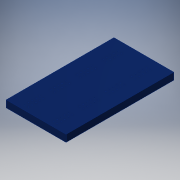
# Autodesk Inventor part: Assembly Plate
Saved by Autodesk Inventor 2019.4 (Build 234330000, 330)
## iProperties
Created: 2021-01-11
Part Number: Assembly Plate
Material: Aluminum, Anodized Blue
Document SubType Name: Modeling
Designer: caleb
Density: 2.7 g/cm^3
Appearance: Anodized - Blue
Author: caleb
Autodesk Inventor part; units mm, degrees
ref_plane "YZ Plane" through (0, 0, 0) normal (1, 0, 0) x (0, 1, 0)
ref_plane "XZ Plane" through (0, 0, 0) normal (0, 1, 0) x (-1, 0, 0)
ref_plane "XY Plane" through (0, 0, 0) normal (0, 0, 1) x (1, 0, 0)
sketch "Sketch1" plane through (0, 0, 0) normal (0, 1, 0) x (-1, 0, 0)
  line L0 (-60, 108) -> (60, 108)
  line L1 (60, 108) -> (60, -108)
  line L2 (60, -108) -> (-60, -108)
  line L3 (-60, -108) -> (-60, 108)
  line L4 (-60, 108) -> (60, -108) construction
  line L5 (60, 108) -> (-60, -108) construction
  point P0 (0, 0)
  dimension "d0" = 120
  dimension "d1" = 216
  constraints: 12 end point, 2 midpoint, 2 parallel, 1 horizontal, 1 perpendicular
  measures "d0" distance of L1.end L2.end
  measures "d1" distance of L0.end L1.end
extrude "Extrusion1" add sketch "Sketch1" along normal blind 14
sketch "Sketch4" plane through (0, 14, 0) normal (0, 1, 0) x (1, 0, 0)
  circle A0 centre (-32.57, -98.05) radius 0.75
  line L0 (-60, 108) -> (-60, -108) projected
  line L1 (-60, -108) -> (60, -108) projected
  circle A1 centre (-32.57, -90.62) radius 0.75
  circle A2 centre (-32.57, -83.19) radius 0.75
  circle A3 centre (-32.57, -75.76) radius 0.75
  circle A4 centre (-32.57, -68.33) radius 0.75
  circle A5 centre (-25.14, -98.05) radius 0.75
  circle A6 centre (-25.14, -90.62) radius 0.75
  circle A7 centre (-25.14, -83.19) radius 0.75
  circle A8 centre (-25.14, -75.76) radius 0.75
  circle A9 centre (-25.14, -68.33) radius 0.75
  circle A10 centre (-32.57, -45.85) radius 0.75
  circle A11 centre (-32.57, -38.42) radius 0.75
  circle A12 centre (-32.57, -30.99) radius 0.75
  circle A13 centre (-32.57, -23.56) radius 0.75
  circle A14 centre (-32.57, -16.13) radius 0.75
  circle A15 centre (-25.14, -45.85) radius 0.75
  circle A16 centre (-25.14, -38.42) radius 0.75
  circle A17 centre (-25.14, -30.99) radius 0.75
  circle A18 centre (-25.14, -23.56) radius 0.75
  circle A19 centre (-25.14, -16.13) radius 0.75
  circle A20 centre (-32.57, 6.35) radius 0.75
  circle A21 centre (-32.57, 13.78) radius 0.75
  circle A22 centre (-32.57, 21.21) radius 0.75
  circle A23 centre (-32.57, 28.64) radius 0.75
  circle A24 centre (-32.57, 36.07) radius 0.75
  circle A25 centre (-25.14, 6.35) radius 0.75
  circle A26 centre (-25.14, 13.78) radius 0.75
  circle A27 centre (-25.14, 21.21) radius 0.75
  circle A28 centre (-25.14, 28.64) radius 0.75
  circle A29 centre (-25.14, 36.07) radius 0.75
  circle A30 centre (-32.57, 58.55) radius 0.75
  circle A31 centre (-32.57, 65.98) radius 0.75
  circle A32 centre (-32.57, 73.41) radius 0.75
  circle A33 centre (-32.57, 80.84) radius 0.75
  circle A34 centre (-32.57, 88.27) radius 0.75
  circle A35 centre (-25.14, 58.55) radius 0.75
  circle A36 centre (-25.14, 65.98) radius 0.75
  circle A37 centre (-25.14, 73.41) radius 0.75
  circle A38 centre (-25.14, 80.84) radius 0.75
  circle A39 centre (-25.14, 88.27) radius 0.75
  circle A40 centre (25.14, -98.05) radius 0.75
  circle A41 centre (25.14, -90.62) radius 0.75
  circle A42 centre (25.14, -83.19) radius 0.75
  circle A43 centre (25.14, -75.76) radius 0.75
  circle A44 centre (25.14, -68.33) radius 0.75
  circle A45 centre (32.57, -98.05) radius 0.75
  circle A46 centre (32.57, -90.62) radius 0.75
  circle A47 centre (32.57, -83.19) radius 0.75
  circle A48 centre (32.57, -75.76) radius 0.75
  circle A49 centre (32.57, -68.33) radius 0.75
  circle A50 centre (25.14, -45.85) radius 0.75
  circle A51 centre (25.14, -38.42) radius 0.75
  circle A52 centre (25.14, -30.99) radius 0.75
  circle A53 centre (25.14, -23.56) radius 0.75
  circle A54 centre (25.14, -16.13) radius 0.75
  circle A55 centre (32.57, -45.85) radius 0.75
  circle A56 centre (32.57, -38.42) radius 0.75
  circle A57 centre (32.57, -30.99) radius 0.75
  circle A58 centre (32.57, -23.56) radius 0.75
  circle A59 centre (32.57, -16.13) radius 0.75
  circle A60 centre (25.14, 6.35) radius 0.75
  circle A61 centre (25.14, 13.78) radius 0.75
  circle A62 centre (25.14, 21.21) radius 0.75
  circle A63 centre (25.14, 28.64) radius 0.75
  circle A64 centre (25.14, 36.07) radius 0.75
  circle A65 centre (32.57, 6.35) radius 0.75
  circle A66 centre (32.57, 13.78) radius 0.75
  circle A67 centre (32.57, 21.21) radius 0.75
  circle A68 centre (32.57, 28.64) radius 0.75
  circle A69 centre (32.57, 36.07) radius 0.75
  circle A70 centre (25.14, 58.55) radius 0.75
  circle A71 centre (25.14, 65.98) radius 0.75
  circle A72 centre (25.14, 73.41) radius 0.75
  circle A73 centre (25.14, 80.84) radius 0.75
  circle A74 centre (25.14, 88.27) radius 0.75
  circle A75 centre (32.57, 58.55) radius 0.75
  circle A76 centre (32.57, 65.98) radius 0.75
  circle A77 centre (32.57, 73.41) radius 0.75
  circle A78 centre (32.57, 80.84) radius 0.75
  circle A79 centre (32.57, 88.27) radius 0.75
  point P0 (0, 0)
  dimension "d31" = 1.5
  dimension "d32" = 27.43
  dimension "d33" = 9.95
  dimension "d36" = 7.43
  dimension "d39" = 7.43
  dimension "d44" = 52.2
  dimension "d47" = 57.71
  constraints: 80 centre point, 2 horizontal, 2 vertical, 158 other
  measures "d31" diameter of A0
  measures "d32" distance from line of L0 A0.centre
  measures "d33" distance from line of L1 A0.centre
  measures "d36" distance of A0.centre A1.centre
  measures "d39" distance of A0.centre A5.centre
  measures "d44" distance of A0.centre A10.centre
  measures "d47" distance of A0.centre A40.centre
extrude "Extrusion3" cut sketch "Sketch4" against normal through all
sketch "Sketch5" plane through (0, 0, 0) normal (0, -1, 0) x (1, 0, 0)
  circle A0 centre (-32.57, -88.27) radius 0.75 projected
  circle A1 centre (-32.57, -80.84) radius 0.75 projected
  circle A2 centre (-32.57, -73.41) radius 0.75 projected
  circle A3 centre (-32.57, -65.98) radius 0.75 projected
  circle A4 centre (-32.57, -58.55) radius 0.75 projected
  circle A5 centre (-25.14, -58.55) radius 0.75 projected
  circle A6 centre (-25.14, -65.98) radius 0.75 projected
  circle A7 centre (-25.14, -73.41) radius 0.75 projected
  circle A8 centre (-25.14, -80.84) radius 0.75 projected
  circle A9 centre (-25.14, -88.27) radius 0.75 projected
  circle A10 centre (-32.57, -88.27) radius 2
  line L0 (-60, 108) -> (-60, -108) projected
  line L1 (-60, -108) -> (60, -108) projected
  circle A11 centre (-32.57, -80.84) radius 2
  circle A12 centre (-32.57, -73.41) radius 2
  circle A13 centre (-32.57, -65.98) radius 2
  circle A14 centre (-32.57, -58.55) radius 2
  circle A15 centre (-25.14, -88.27) radius 2
  circle A16 centre (-25.14, -80.84) radius 2
  circle A17 centre (-25.14, -73.41) radius 2
  circle A18 centre (-25.14, -65.98) radius 2
  circle A19 centre (-25.14, -58.55) radius 2
  circle A20 centre (-25.14, -13.78) radius 2
  circle A21 centre (-32.57, -6.35) radius 2
  circle A22 centre (-32.57, -21.21) radius 2
  circle A23 centre (-25.14, -28.64) radius 2
  circle A24 centre (-25.14, -36.07) radius 2
  circle A25 centre (-25.14, -6.35) radius 2
  circle A26 centre (-32.57, -36.07) radius 2
  circle A27 centre (-32.57, -28.64) radius 2
  circle A28 centre (-25.14, -21.21) radius 2
  circle A29 centre (-32.57, -13.78) radius 2
  circle A30 centre (-25.14, 38.42) radius 2
  circle A31 centre (-32.57, 45.85) radius 2
  circle A32 centre (-32.57, 30.99) radius 2
  circle A33 centre (-25.14, 23.56) radius 2
  circle A34 centre (-25.14, 16.13) radius 2
  circle A35 centre (-25.14, 45.85) radius 2
  circle A36 centre (-32.57, 16.13) radius 2
  circle A37 centre (-32.57, 23.56) radius 2
  circle A38 centre (-25.14, 30.99) radius 2
  circle A39 centre (-32.57, 38.42) radius 2
  circle A40 centre (-25.14, 90.62) radius 2
  circle A41 centre (-32.57, 98.05) radius 2
  circle A42 centre (-32.57, 83.19) radius 2
  circle A43 centre (-25.14, 75.76) radius 2
  circle A44 centre (-25.14, 68.33) radius 2
  circle A45 centre (-25.14, 98.05) radius 2
  circle A46 centre (-32.57, 68.33) radius 2
  circle A47 centre (-32.57, 75.76) radius 2
  circle A48 centre (-25.14, 83.19) radius 2
  circle A49 centre (-32.57, 90.62) radius 2
  circle A50 centre (32.57, -65.98) radius 2
  circle A51 centre (25.14, -58.55) radius 2
  circle A52 centre (25.14, -73.41) radius 2
  circle A53 centre (32.57, -80.84) radius 2
  circle A54 centre (32.57, -88.27) radius 2
  circle A55 centre (32.57, -58.55) radius 2
  circle A56 centre (25.14, -88.27) radius 2
  circle A57 centre (25.14, -80.84) radius 2
  circle A58 centre (32.57, -73.41) radius 2
  circle A59 centre (25.14, -65.98) radius 2
  circle A60 centre (32.57, -13.78) radius 2
  circle A61 centre (25.14, -6.35) radius 2
  circle A62 centre (25.14, -21.21) radius 2
  circle A63 centre (32.57, -28.64) radius 2
  circle A64 centre (32.57, -36.07) radius 2
  circle A65 centre (32.57, -6.35) radius 2
  circle A66 centre (25.14, -36.07) radius 2
  circle A67 centre (25.14, -28.64) radius 2
  circle A68 centre (32.57, -21.21) radius 2
  circle A69 centre (25.14, -13.78) radius 2
  circle A70 centre (32.57, 38.42) radius 2
  circle A71 centre (25.14, 45.85) radius 2
  circle A72 centre (25.14, 30.99) radius 2
  circle A73 centre (32.57, 23.56) radius 2
  circle A74 centre (32.57, 16.13) radius 2
  circle A75 centre (32.57, 45.85) radius 2
  circle A76 centre (25.14, 16.13) radius 2
  circle A77 centre (25.14, 23.56) radius 2
  circle A78 centre (32.57, 30.99) radius 2
  circle A79 centre (25.14, 38.42) radius 2
  circle A80 centre (32.57, 90.62) radius 2
  circle A81 centre (25.14, 98.05) radius 2
  circle A82 centre (25.14, 83.19) radius 2
  circle A83 centre (32.57, 75.76) radius 2
  circle A84 centre (32.57, 68.33) radius 2
  circle A85 centre (32.57, 98.05) radius 2
  circle A86 centre (25.14, 68.33) radius 2
  circle A87 centre (25.14, 75.76) radius 2
  circle A88 centre (32.57, 83.19) radius 2
  circle A89 centre (25.14, 90.62) radius 2
  point P0 (0, 0)
  point P1 (-25.14, -13.78)
  point P2 (-32.57, -13.78)
  point P3 (-25.14, -21.21)
  point P4 (-32.57, -21.21)
  point P5 (-25.14, -6.35)
  point P6 (-25.14, 38.42)
  point P7 (-32.57, 38.42)
  point P8 (-25.14, 30.99)
  point P9 (-32.57, 30.99)
  point P10 (-25.14, 45.85)
  point P11 (-25.14, 90.62)
  point P12 (-25.14, 83.19)
  point P13 (-32.57, 83.19)
  point P14 (-25.14, 98.05)
  point P15 (32.57, -65.98)
  point P16 (25.14, -65.98)
  point P17 (32.57, -73.41)
  point P18 (25.14, -73.41)
  point P19 (25.14, -58.55)
  point P20 (32.57, -58.55)
  point P21 (32.57, -13.78)
  point P22 (25.14, -13.78)
  point P23 (32.57, -21.21)
  point P24 (25.14, -21.21)
  point P25 (25.14, -6.35)
  point P26 (32.57, -6.35)
  point P27 (32.57, 38.42)
  point P28 (25.14, 38.42)
  point P29 (32.57, 30.99)
  point P30 (25.14, 30.99)
  point P31 (25.14, 45.85)
  point P32 (32.57, 45.85)
  point P33 (32.57, 90.62)
  point P34 (25.14, 90.62)
  point P35 (32.57, 83.19)
  point P36 (25.14, 83.19)
  point P37 (25.14, 98.05)
  point P38 (32.57, 98.05)
  dimension "d52" = 4
  dimension "d55" = 7.43
  dimension "d58" = 7.43
  dimension "d63" = 52.2
  dimension "d66" = 57.71
  constraints: 80 centre point, 80 coincident, 2 horizontal, 2 vertical, 300 other
  measures "d52" diameter of A10
  measures "d55" distance of A0.centre point (-32.57, -80.84)
  measures "d58" distance of A0.centre point (-25.14, -88.27)
  measures "d63" distance of A18.centre A20.centre
  measures "d66" distance of A18.centre A50.centre
extrude "Extrusion4" cut sketch "Sketch5" against normal blind 12
sketch "Sketch6" plane through (0, 0, 0) normal (0, -1, 0) x (1, 0, 0)
  line L0 (42.5, -100.5) -> (-42.5, -100.5)
  line L1 (-52.5, -90.5) -> (-52.5, 90.5)
  line L2 (-42.5, 100.5) -> (42.5, 100.5)
  line L3 (52.5, 90.5) -> (52.5, -90.5)
  line L4 (52.5, -100.5) -> (-52.5, 100.5) construction
  line L5 (-52.5, -100.5) -> (52.5, 100.5) construction
  line L6 (-60, 108) -> (-60, -108) projected
  line L7 (60, 108) -> (-60, 108) projected
  arc A0 (-52.5, -90.5) -> (-42.5, -100.5) centre (-42.5, -90.5) ccw
  arc A1 (42.5, -100.5) -> (52.5, -90.5) centre (42.5, -90.5) ccw
  arc A2 (52.5, 90.5) -> (42.5, 100.5) centre (42.5, 90.5) ccw
  arc A3 (-42.5, 100.5) -> (-52.5, 90.5) centre (-42.5, 90.5) ccw
  point P0 (0, 0)
  dimension "d71" = 7.5
  dimension "d72" = 7.5
  dimension "d73" = 10
  constraints: 12 end point, 8 point on circle, 8 point on line, 8 tangent, 4 centre point, 3 equal radius, 2 midpoint, 2 parallel, 1 horizontal, 1 perpendicular
  measures "d71" distance between parallel lines of L7 L2
  measures "d72" distance between parallel lines of L6 L1
  measures "d73" radius of A0
extrude "Extrusion5" cut sketch "Sketch6" against normal blind 5
body "Solid1"
